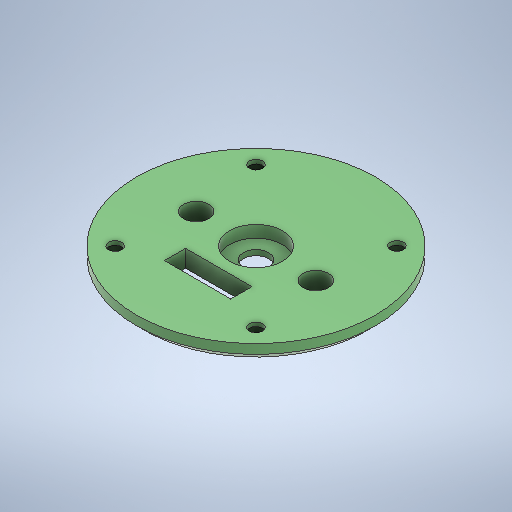
# Autodesk Inventor part: SCARA swivel top - lid
Saved by Autodesk Inventor 2025.2 (Build 292293000, 293)
## iProperties
Created: 2025-01-27
Part Number: SCARA swivel top - lid
Material: Generic
Document SubType Name: Modeling
Designer: caomi
Density: 1 g/cm^3
Appearance: Default
Author: caomi
Autodesk Inventor part; units mm, degrees
ref_plane "YZ Plane" through (0, 0, 0) normal (1, 0, 0) x (0, 1, 0)
ref_plane "XZ Plane" through (0, 0, 0) normal (0, 1, 0) x (-1, 0, 0)
ref_plane "XY Plane" through (0, 0, 0) normal (0, 0, 1) x (1, 0, 0)
sketch "Sketch1" plane through (0, 0, 0) normal (0, 1, 0) x (-1, 0, 0)
  circle A0 centre (0, 0) radius 45
  circle A1 centre (0, 0) radius 10
  circle A2 centre (22.5, 0) radius 4.75
  circle A3 centre (-22.5, 0) radius 4.75
  line L0 (0, -25.6154) -> (0, 19.3488) construction
  circle A4 centre (0, 0) radius 4.75
  line L1 (12.5, 22) -> (-12.5, 22)
  line L2 (-12.5, 22) -> (-12.5, 14)
  line L3 (-12.5, 14) -> (12.5, 14)
  line L4 (12.5, 14) -> (12.5, 22)
  line L5 (12.5, 22) -> (-12.5, 14) construction
  line L6 (-12.5, 22) -> (12.5, 14) construction
  point P0 (0, 18)
  dimension "d0" = 90
  dimension "d1" = 20
  dimension "d2" = 45
  dimension "d20" = 18
  dimension "d21" = 8
  dimension "d22" = 25
  dimension "d26" = 9.5
  constraints: 14 end point, 5 centre point, 3 coincident, 2 equal radius, 2 midpoint, 2 parallel, 2 point on line, 1 horizontal, 1 horizontal alignment, 1 perpendicular, 1 vertical, 1 other
  measures "d0" diameter of A0
  measures "d1" diameter of A1
  measures "d2" distance of A3.centre A2.centre
  measures "d20" distance of point (0, 0) point (0, 18)
  measures "d21" distance of L1.end L2.end
  measures "d22" distance of L1.start L1.end
  measures "d26" diameter of A4
extrude "Extrusion1" add sketch "Sketch1" against normal blind 2 contours A0 | A1
extrude "Extrusion2" add sketch "Sketch1" along normal blind 4.5 contours A0
sketch "Sketch2" plane through (0, -2, 0) normal (0, -1, 0) x (1, 0, 0)
  line L0 (26.5165, -26.5165) -> (0, 0) construction
  line L1 (17.2429, 0) -> (-14.3285, 0) construction
  line L2 (0, -10.0849) -> (0, 10.0849) construction
  point P0 (-26.5165, -26.5165)
  point P1 (26.5165, 26.5165)
  point P2 (-26.5165, 26.5165)
  dimension "d9" = 37.5
  dimension "d10" = 45
  constraints: 6 end point, 3 symmetric about line, 2 midpoint, 2 point on line, 1 coincident, 1 horizontal, 1 vertical
  measures "d9" distance of L0.start L0.end
  measures "d10" angle of L0 L1
hole "Hole1" at (26.5165, -2, -26.5165) at (-26.5165, -2, -26.5165) at (26.5165, -2, 26.5165) at (-26.5165, -2, 26.5165) direction (0, 1, 0) diameter 5 end through all counterbore diameter 7.2 counterbore depth 5
chamfer "Chamfer1" distance 3 angle 45 1 edges at (45, -2, 0)
body "Solid1"
